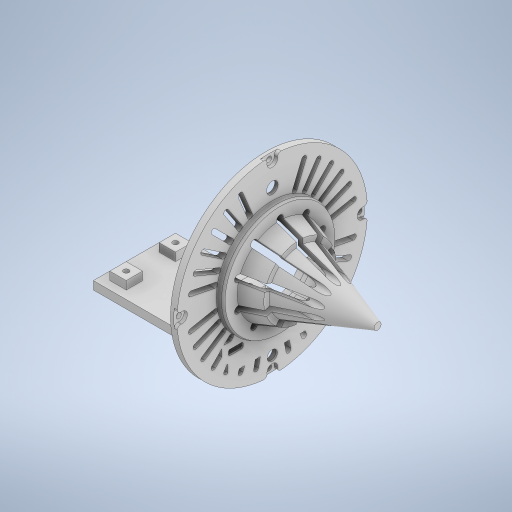
# Autodesk Inventor part: Temp_controller_trent_back
Saved by Autodesk Inventor 2024 (Build 280153000, 153)
## iProperties
Created: 2026-04-14
Part Number: Temp_controller_trent_back
Material: Generic
Document SubType Name: Modeling
Designer: Péter
Density: 1 g/cm^3
Appearance: Default
Author: Péter
Autodesk Inventor part; units mm, degrees
ref_plane "YZ Plane" through (0, 0, 0) normal (1, 0, 0) x (0, 1, 0)
ref_plane "XZ Plane" through (0, 0, 0) normal (0, 1, 0) x (-1, 0, 0)
ref_plane "XY Plane" through (0, 0, 0) normal (0, 0, 1) x (1, 0, 0)
sketch "Sketch1" plane through (0, 0, 0) normal (1, 0, 0) x (0, 1, 0)
  circle A0 centre (0, 0) radius 58
  dimension "d0" = 116
  constraints: 1 centre point, 1 coincident
  measures "d0" diameter of A0
extrude "Extrusion1" add sketch "Sketch1" along normal blind 4
sketch "Sketch2" plane through (0, 0, 0) normal (-1, 0, 0) x (0, 0, 1)
  line L0 (-25, -37.5) -> (25, -37.5)
  line L1 (25, -37.5) -> (25, -42.5)
  line L2 (25, -42.5) -> (-25, -42.5)
  line L3 (-25, -42.5) -> (-25, -37.5)
  line L4 (-25, -37.5) -> (25, -42.5) construction
  line L5 (25, -37.5) -> (-25, -42.5) construction
  point P0 (0, 0)
  point P1 (0, -40)
  dimension "d3" = 50
  dimension "d4" = 5
  dimension "d5" = 0
  dimension "d6" = 40
  constraints: 12 end point, 2 midpoint, 2 parallel, 1 horizontal, 1 perpendicular
  measures "d3" distance of L1.end L2.end
  measures "d4" distance of L0.end L1.end
  measures "d5" horizontal distance of point (0, 0) point (0, -40)
  measures "d6" distance of point (0, 0) point (0, -40)
extrude "Extrusion2" add sketch "Sketch2" along normal blind 80
sketch "Sketch3" plane through (0, -37.5, 25) normal (0, 1, 0) x (1, 0, 0)
  line L0 (-20, 45) -> (-30, 45)
  line L1 (-30, 45) -> (-30, 35)
  line L2 (-30, 35) -> (-20, 35)
  line L3 (-20, 35) -> (-20, 45)
  line L4 (-20, 45) -> (-30, 35) construction
  line L5 (-30, 45) -> (-20, 35) construction
  line L6 (-20, 15) -> (-30, 15)
  line L7 (-30, 15) -> (-30, 5)
  line L8 (-30, 5) -> (-20, 5)
  line L9 (-20, 5) -> (-20, 15)
  line L10 (-20, 15) -> (-30, 5) construction
  line L11 (-30, 15) -> (-20, 5) construction
  line L12 (-75, 35) -> (-65, 35)
  line L13 (-65, 35) -> (-65, 45)
  line L14 (-65, 45) -> (-75, 45)
  line L15 (-75, 45) -> (-75, 35)
  line L16 (-75, 35) -> (-65, 45) construction
  line L17 (-65, 35) -> (-75, 45) construction
  line L18 (-75, 15) -> (-65, 15)
  line L19 (-65, 15) -> (-65, 5)
  line L20 (-65, 5) -> (-75, 5)
  line L21 (-75, 5) -> (-75, 15)
  line L22 (-75, 15) -> (-65, 5) construction
  line L23 (-65, 15) -> (-75, 5) construction
  line L24 (-25, 40) -> (-70, 40) construction
  line L25 (-70, 40) -> (-70, 10) construction
  line L26 (-25, 10) -> (-70, 10) construction
  line L27 (-25, 10) -> (-25, 40) construction
  line L28 (0, 50) -> (0, 0) projected
  line L29 (0, 50) -> (-80, 50) projected
  line L30 (-80, 0) -> (-80, 50) projected
  point P0 (0, 25)
  point P1 (-80, 25)
  dimension "d9" = 10
  dimension "d10" = 10
  dimension "d11" = 10
  dimension "d12" = 10
  dimension "d13" = 10
  dimension "d14" = 10
  dimension "d15" = 10
  dimension "d16" = 10
  dimension "d17" = 30
  dimension "d18" = 45
  dimension "d19" = 15
  dimension "d20" = 10
  constraints: 56 end point, 12 parallel, 9 midpoint, 5 horizontal, 5 perpendicular
  measures "d9" distance of L2.end L1.end
  measures "d10" distance of L1.end L0.end
  measures "d11" distance of L8.end L7.end
  measures "d12" distance of L7.end L6.end
  measures "d13" distance of L14.end L13.end
  measures "d14" distance of L13.end L12.end
  measures "d15" distance of L19.end L20.end
  measures "d16" distance of L18.end L19.end
  measures "d17" distance of L24.end L25.end
  measures "d18" distance of L24.start L24.end
  measures "d19" distance from line of point (-80, 25) L24
  measures "d20" distance between parallel lines of L30 L25
extrude "Extrusion3" add sketch "Sketch3" along normal blind 5
sketch "Sketch4" plane through (0, -32.5, 25) normal (0, 1, 0) x (1, 0, 0)
  line L0 (-25, 10) -> (-25, 40) construction
  line L1 (-25, 40) -> (-70, 40) construction
  line L2 (-70, 40) -> (-70, 10) construction
  line L3 (-70, 10) -> (-25, 10) construction
  line L4 (0, 50) -> (-80, 50) projected
  line L5 (-80, 0) -> (-80, 50) projected
  line L6 (-75, 15) -> (-75, 5) projected
  line L7 (-75, 5) -> (-65, 5) projected
  point P0 (0, 25)
  dimension "d23" = 45
  dimension "d24" = 30
  dimension "d25" = 5
  dimension "d26" = 5
  constraints: 8 end point, 4 parallel, 1 vertical
  measures "d23" distance of L0.end L1.end
  measures "d24" distance of L1.end L2.end
  measures "d25" distance between parallel lines of L6 L2
  measures "d26" distance between parallel lines of L7 L3
hole "Hole1" at (-25, -32.5, -15) at (-25, -32.5, 15) at (-70, -32.5, 15) at (-70, -32.5, -15) direction (0, -1, 0) diameter 3.2 end through all
sketch "Sketch5" plane through (0, -42.5, -25) normal (0, -1, 0) x (1, 0, 0)
  circle A0 centre (-70, 40) radius 1.6 projected
  line L0 (-68.3834, 37.2) -> (-71.6166, 37.2)
  line L1 (-71.6166, 37.2) -> (-73.2332, 40)
  line L2 (-73.2332, 40) -> (-71.6166, 42.8)
  line L3 (-71.6166, 42.8) -> (-68.3834, 42.8)
  line L4 (-68.3834, 42.8) -> (-66.7668, 40)
  line L5 (-66.7668, 40) -> (-68.3834, 37.2)
  circle A1 centre (-70, 10) radius 1.6 projected
  line L6 (-68.3834, 7.2) -> (-71.6166, 7.2)
  line L7 (-71.6166, 7.2) -> (-73.2332, 10)
  line L8 (-73.2332, 10) -> (-71.6166, 12.8)
  line L9 (-71.6166, 12.8) -> (-68.3834, 12.8)
  line L10 (-68.3834, 12.8) -> (-66.7668, 10)
  line L11 (-66.7668, 10) -> (-68.3834, 7.2)
  line L12 (0, 50) -> (-80, 50) projected
  line L13 (0, 0) -> (-80, 0) projected
  line L14 (-23.3834, 37.2) -> (-26.6166, 37.2)
  line L15 (-26.6166, 37.2) -> (-28.2332, 40)
  line L16 (-28.2332, 40) -> (-26.6166, 42.8)
  line L17 (-26.6166, 42.8) -> (-23.3834, 42.8)
  line L18 (-23.3834, 42.8) -> (-21.7668, 40)
  line L19 (-21.7668, 40) -> (-23.3834, 37.2)
  circle A2 centre (-25, 10) radius 1.6 projected
  line L20 (-23.3834, 12.8) -> (-21.7668, 10)
  line L21 (-21.7668, 10) -> (-23.3834, 7.2)
  line L22 (-23.3834, 7.2) -> (-26.6166, 7.2)
  line L23 (-26.6166, 7.2) -> (-28.2332, 10)
  line L24 (-28.2332, 10) -> (-26.6166, 12.8)
  line L25 (-26.6166, 12.8) -> (-23.3834, 12.8)
  point P0 (0, 25)
  point P1 (-70, 40)
  point P2 (-70, 10)
  point P3 (-25, 40)
  point P4 (-25, 10)
  point P5 (-25, 37.2)
  dimension "d34" = 5.6
  dimension "d35" = 5.6
  dimension "d36" = 5.6
  dimension "d37" = 5.6
  constraints: 48 end point, 4 parallel, 3 coincident, 1 midpoint, 52 other
  measures "d34" distance from line of point (-25, 37.2) L17
  measures "d35" distance between parallel lines of L3 L0
  measures "d36" distance between parallel lines of L6 L9
  measures "d37" distance between parallel lines of L22 L25
extrude "Extrusion4" cut sketch "Sketch5" against normal blind 5
sketch "Sketch6" plane through (0, 0, 0) normal (0, 0, 1) x (1, 0, 0)
  line L0 (4, -58) -> (4, 58) projected
  line L1 (4, 34.1056) -> (7.1617, 34.1056)
  line L2 (7.1617, 34.1056) -> (8.6675, 33.4211)
  line L3 (8.6675, 33.4211) -> (8.6675, 26.0286)
  line L4 (8.6675, 26.0286) -> (20.6939, 21.84)
  line L5 (20.6939, 21.84) -> (20.6939, 18.6633)
  line L6 (20.6939, 18.6633) -> (68.159, 2.1319)
  line L7 (68.159, 2.1319) -> (68.159, 0)
  line L8 (68.159, 0) -> (65.159, 0)
  line L9 (65.159, 0) -> (17.6939, 16.5314)
  line L10 (17.6939, 16.5314) -> (17.6939, 19.7081)
  line L11 (17.6939, 19.7081) -> (6.6667, 23.5487)
  line L12 (6.6667, 23.5487) -> (4, 23.5487)
  line L13 (-109.6318, 0) -> (97.7908, 0) projected
  line L14 (59.0379, 2.1319) -> (59.0379, 0)
  line L15 (65.159, 0) -> (59.0379, 0)
  point P0 (0, 0)
  point P1 (20.6939, 20.2516)
  dimension "d53" = 0
  dimension "d54" = 3
  dimension "d55" = 3
  dimension "d56" = 3
  dimension "d57" = 3
  constraints: 28 end point, 6 parallel, 6 point on line, 3 perpendicular, 1 horizontal, 1 midpoint
  measures "d53" distance from line of point (0, 0) L8
  measures "d54" distance between parallel lines of L4 L11
  measures "d55" distance from line of point (20.694, 20.252) L10
  measures "d56" distance between parallel lines of L9 L6
  measures "d57" distance from line of L8.end L7
revolve "Revolution1" add sketch "Sketch6" angle 360 about axis through (-10, 0, 0) along (1, 0, 0) contours L0 L1 L2 L3 L4 L5 L6 L7 L8 L9 L10 L11 L12 | L14 L9 L13
sketch "Sketch7" plane through (0, 0, 0) normal (-1, 0, 0) x (0, 0, 1)
  circle A0 centre (0, 0) radius 23.5
  dimension "d59" = 47
  constraints: 1 centre point, 1 coincident
  measures "d59" diameter of A0
extrude "Extrusion5" cut sketch "Sketch7" against normal up to surface (4 mm away)
sketch "Sketch9" plane through (68.159, 0, 0) normal (1, 0, 0) x (0, 0, -1)
  line L0 (0, 27) -> (0, 12) construction
  line L1 (-2, 27) -> (-2, 12)
  line L2 (2, 12) -> (2, 27)
  arc A0 (2, 27) -> (-2, 27) centre (0, 27) ccw
  arc A1 (-2, 12) -> (2, 12) centre (0, 12) ccw
  line L3 (-15.8702, 21.8435) -> (-7.0534, 9.7082) construction
  line L4 (-17.4882, 20.6679) -> (-8.6715, 8.5326)
  line L5 (-5.4354, 10.8838) -> (-14.2522, 23.019)
  arc A2 (-14.2522, 23.019) -> (-17.4882, 20.6679) centre (-15.8702, 21.8435) ccw
  arc A3 (-8.6715, 8.5326) -> (-5.4354, 10.8838) centre (-7.0534, 9.7082) ccw
  line L6 (-25.6785, 8.3435) -> (-11.4127, 3.7082) construction
  line L7 (-26.2966, 6.4413) -> (-12.0307, 1.8061)
  line L8 (-10.7946, 5.6103) -> (-25.0605, 10.2456)
  arc A4 (-25.0605, 10.2456) -> (-26.2966, 6.4413) centre (-25.6785, 8.3435) ccw
  arc A5 (-12.0307, 1.8061) -> (-10.7946, 5.6103) centre (-11.4127, 3.7082) ccw
  line L9 (-25.6785, -8.3435) -> (-11.4127, -3.7082) construction
  line L10 (-25.0605, -10.2456) -> (-10.7946, -5.6103)
  line L11 (-12.0307, -1.8061) -> (-26.2966, -6.4413)
  arc A6 (-26.2966, -6.4413) -> (-25.0605, -10.2456) centre (-25.6785, -8.3435) ccw
  arc A7 (-10.7946, -5.6103) -> (-12.0307, -1.8061) centre (-11.4127, -3.7082) ccw
  line L12 (-15.8702, -21.8435) -> (-7.0534, -9.7082) construction
  line L13 (-14.2522, -23.019) -> (-5.4354, -10.8838)
  line L14 (-8.6715, -8.5326) -> (-17.4882, -20.6679)
  arc A8 (-17.4882, -20.6679) -> (-14.2522, -23.019) centre (-15.8702, -21.8435) ccw
  arc A9 (-5.4354, -10.8838) -> (-8.6715, -8.5326) centre (-7.0534, -9.7082) ccw
  line L15 (0, -27) -> (0, -12) construction
  line L16 (2, -27) -> (2, -12)
  line L17 (-2, -12) -> (-2, -27)
  arc A10 (-2, -27) -> (2, -27) centre (0, -27) ccw
  arc A11 (2, -12) -> (-2, -12) centre (0, -12) ccw
  line L18 (15.8702, -21.8435) -> (7.0534, -9.7082) construction
  line L19 (17.4882, -20.6679) -> (8.6715, -8.5326)
  line L20 (5.4354, -10.8838) -> (14.2522, -23.019)
  arc A12 (14.2522, -23.019) -> (17.4882, -20.6679) centre (15.8702, -21.8435) ccw
  arc A13 (8.6715, -8.5326) -> (5.4354, -10.8838) centre (7.0534, -9.7082) ccw
  line L21 (25.6785, -8.3435) -> (11.4127, -3.7082) construction
  line L22 (26.2966, -6.4413) -> (12.0307, -1.8061)
  line L23 (10.7946, -5.6103) -> (25.0605, -10.2456)
  arc A14 (25.0605, -10.2456) -> (26.2966, -6.4413) centre (25.6785, -8.3435) ccw
  arc A15 (12.0307, -1.8061) -> (10.7946, -5.6103) centre (11.4127, -3.7082) ccw
  line L24 (25.6785, 8.3435) -> (11.4127, 3.7082) construction
  line L25 (25.0605, 10.2456) -> (10.7946, 5.6103)
  line L26 (12.0307, 1.8061) -> (26.2966, 6.4413)
  arc A16 (26.2966, 6.4413) -> (25.0605, 10.2456) centre (25.6785, 8.3435) ccw
  arc A17 (10.7946, 5.6103) -> (12.0307, 1.8061) centre (11.4127, 3.7082) ccw
  line L27 (15.8702, 21.8435) -> (7.0534, 9.7082) construction
  line L28 (14.2522, 23.019) -> (5.4354, 10.8838)
  line L29 (8.6715, 8.5326) -> (17.4882, 20.6679)
  arc A18 (17.4882, 20.6679) -> (14.2522, 23.019) centre (15.8702, 21.8435) ccw
  arc A19 (5.4354, 10.8838) -> (8.6715, 8.5326) centre (7.0534, 9.7082) ccw
  point P0 (0, 0)
  point P1 (0, 19.5)
  point P2 (-11.4618, 15.7758)
  point P3 (-18.5456, 6.0258)
  point P4 (-18.5456, -6.0258)
  point P5 (-11.4618, -15.7758)
  point P6 (0, -19.5)
  point P7 (11.4618, -15.7758)
  point P8 (18.5456, -6.0258)
  point P9 (18.5456, 6.0258)
  point P10 (11.4618, 15.7758)
  dimension "d70" = 15
  dimension "d71" = 4
  dimension "d72" = 12
  dimension "d75" = 360
  constraints: 80 end point, 40 point on circle, 20 centre point, 4 tangent, 1 midpoint, 1 parallel, 1 vertical, 121 other
  measures "d70" distance of L0.start L0.end
  measures "d71" diameter of A1
  measures "d72" distance of point (0, 0) L0.end
extrude "Extrusion7" cut sketch "Sketch9" against normal up to surface (68.159 mm away)
sketch "Sketch10" plane through (4, 0, 0) normal (1, 0, 0) x (0, 0, -1)
  point P0 (0, 0)
  point P1 (0, -55)
  dimension "d79" = 55
  measures "d79" distance of point (0, 0) point (0, -55)
hole "Hole2" at (4, -55, 0) direction (-1, 0, 0) diameter 3.2 end through all
pattern_circular "Circular Pattern1" count 4 over 360 about axis through (5.5808, 0, 0) along (1, 0, 0) of "Hole2"
sketch "Sketch11" plane through (0, 0, 0) normal (-1, 0, 0) x (0, 0, 1)
  line L0 (-32.5, -29.5) -> (-12, -29.5)
  line L1 (-12, -29.5) -> (-12, -36.5)
  line L2 (-12, -36.5) -> (-32.5, -36.5)
  line L3 (-32.5, -36.5) -> (-32.5, -29.5)
  line L4 (-25, -37.5) -> (25, -37.5) projected
  point P0 (0, 0)
  dimension "d90" = 20.5
  dimension "d91" = 7
  dimension "d92" = 12
  dimension "d107" = 1
  constraints: 8 end point, 2 parallel, 1 horizontal, 1 perpendicular
  measures "d90" distance of L0.start L0.end
  measures "d91" distance of L2.end L0.start
  measures "d92" distance from line of point (0, 0) L1
  measures "d107" distance between parallel lines of L4 L2
extrude "Extrusion8" cut sketch "Sketch11" against normal blind 3
sketch "Sketch12" plane through (3, 0, 0) normal (-1, 0, 0) x (0, 0, 1)
  line L0 (-14.25, -33) -> (-30.25, -33) construction
  line L1 (-32.5, -29.5) -> (-12, -29.5) projected
  point P0 (0, 0)
  point P1 (-22.25, -29.5)
  point P2 (-22.25, -33)
  dimension "d96" = 16
  dimension "d97" = 3.5
  dimension "d98" = 0
  constraints: 2 end point, 2 midpoint, 1 parallel
  measures "d96" distance of L0.start L0.end
  measures "d97" distance between parallel lines of L1 L0
  measures "d98" horizontal distance of point (-22.25, -29.5) point (-22.25, -33)
hole "Hole3" at (3, -33, -30.25) at (3, -33, -14.25) direction (1, 0, 0) diameter 2.1 end through all
sketch "Sketch13" plane through (3, 0, 0) normal (-1, 0, 0) x (0, 0, 1)
  line L0 (-25.75, -31.35) -> (-18.75, -31.35)
  line L1 (-17.75, -32.35) -> (-17.75, -33.65)
  line L2 (-18.75, -34.65) -> (-25.75, -34.65)
  line L3 (-26.75, -33.65) -> (-26.75, -32.35)
  circle A0 centre (-30.25, -33) radius 1.05 projected
  arc A1 (-25.75, -31.35) -> (-26.75, -32.35) centre (-25.75, -32.35) ccw
  arc A2 (-26.75, -33.65) -> (-25.75, -34.65) centre (-25.75, -33.65) ccw
  arc A3 (-17.75, -32.35) -> (-18.75, -31.35) centre (-18.75, -32.35) ccw
  arc A4 (-18.75, -34.65) -> (-17.75, -33.65) centre (-18.75, -33.65) ccw
  point P0 (0, 0)
  point P1 (-17.75, -34.65)
  point P2 (-17.75, -31.35)
  point P3 (-26.75, -34.65)
  point P4 (-22.25, -34.65)
  point P5 (-26.75, -33)
  dimension "d108" = 9
  dimension "d109" = 3.3
  dimension "d110" = 8
  dimension "d111" = 0
  dimension "d112" = 1
  dimension "d113" = 1
  constraints: 8 end point, 8 point on circle, 8 tangent, 6 point on line, 4 centre point, 2 equal radius, 2 midpoint, 2 parallel, 1 horizontal, 1 perpendicular
  measures "d108" distance of point (-17.75, -34.65) point (-26.75, -34.65)
  measures "d109" distance of point (-17.75, -31.35) point (-17.75, -34.65)
  measures "d110" horizontal distance of A0.centre point (-22.25, -34.65)
  measures "d111" vertical distance of point (-26.75, -33) A0.centre
  measures "d112" radius of A1
  measures "d113" radius of A2
extrude "Extrusion9" cut sketch "Sketch13" against normal up to surface (1 mm away) contours L0 A3 L1 A4 L2 A2 L3 A1
mirror "Mirror1" about plane through (0, 0, 0) normal (0, 0, 1) of "Extrusion9"
sketch "Sketch14" plane through (3, -33.65, 17.75) normal (1, 0, 0) x (0, 0, -1)
  line L0 (-8, 2.3) -> (-1, 2.3)
  line L1 (0, 1.3) -> (0, 0)
  line L2 (-1, -1) -> (-8, -1)
  line L3 (-9, 0) -> (-9, 1.3)
  line L4 (-8, 2.3) -> (-1, 2.3) projected
  line L5 (-9, 0) -> (-9, 1.3) projected
  line L6 (0, 1.3) -> (0, 0) projected
  line L7 (-1, -1) -> (-8, -1) projected
  arc A0 (-8, 2.3) -> (-9, 1.3) centre (-8, 1.3) ccw
  arc A1 (-9, 0) -> (-8, -1) centre (-8, 0) ccw
  arc A2 (-1, -1) -> (0, 0) centre (-1, 0) ccw
  arc A3 (0, 1.3) -> (-1, 2.3) centre (-1, 1.3) ccw
  point P0 (17.75, 33.65)
  dimension "d116" = 1
  constraints: 8 end point, 8 point on circle, 8 tangent, 4 centre point, 4 collinear, 3 equal radius, 2 parallel, 1 horizontal, 1 perpendicular
  measures "d116" radius of A0
extrude "Extrusion10" cut sketch "Sketch14" against normal up to surface (3 mm away)
sketch "Sketch15" plane through (0, 0, 0) normal (-1, 0, 0) x (0, 0, 1)
  line L0 (15.75, -29.35) -> (28.75, -29.35)
  line L1 (28.75, -29.35) -> (28.75, -36.65)
  line L2 (28.75, -36.65) -> (15.75, -36.65)
  line L3 (15.75, -36.65) -> (15.75, -29.35)
  line L4 (18.75, -31.35) -> (25.75, -31.35) projected
  line L5 (26.75, -32.35) -> (26.75, -33.65) projected
  line L6 (17.75, -33.65) -> (17.75, -32.35) projected
  line L7 (25.75, -34.65) -> (18.75, -34.65) projected
  point P0 (0, 0)
  point P1 (26.75, -33)
  point P2 (15.75, -33)
  dimension "d119" = 2
  dimension "d120" = 2
  dimension "d121" = 2
  dimension "d122" = 2
  constraints: 8 end point, 2 midpoint, 2 parallel, 1 horizontal, 1 perpendicular
  measures "d119" distance between parallel lines of L0 L4
  measures "d120" distance from line of point (26.75, -33) L1
  measures "d121" distance from line of point (15.75, -33) L6
  measures "d122" distance between parallel lines of L7 L2
extrude "Extrusion11" cut sketch "Sketch15" against normal blind 3
ref_plane "Work Plane1" through (4, -36.25, 25.75) normal (0, 1, 0) x (1, 0, 0)
sketch "Sketch16" plane through (4, -36.25, 25.75) normal (0, 1, 0) x (1, 0, 0)
  line L0 (-7, 0.75) -> (-10, 0.75)
  line L1 (-10, 0.75) -> (-10, 8.5)
  line L2 (-10, 8.5) -> (-7, 8.5)
  line L3 (-7, 8.5) -> (-7, 0.75)
  line L4 (-4, 50.75) -> (-4, 0.75) projected
  line L5 (-4, 10) -> (-1, 10) projected
  line L6 (-4, 0.75) -> (-84, 0.75) projected
  line L7 (-7, 0.75) -> (-10, 0.75)
  point P0 (-4, 25.75)
  dimension "d126" = 3
  dimension "d128" = 3
  dimension "d129" = 1.5
  constraints: 10 end point, 4 point on line, 2 parallel, 1 collinear, 1 horizontal, 1 perpendicular
  measures "d126" distance of L1.end L2.end
  measures "d128" distance between parallel lines of L4 L3
  measures "d129" distance between parallel lines of L5 L2
extrude "Extrusion12" add sketch "Sketch16" against normal up to surface (1.25 mm away)
sketch "Sketch18" plane through (0, 0, 0) normal (-1, 0, 0) x (0, 0, 1)
  circle A0 centre (0, -47.5) radius 4.25
  line L0 (25, -42.5) -> (-25, -42.5) projected
  point P0 (0, 0)
  dimension "d133" = 8.5
  dimension "d134" = 5
  constraints: 1 centre point
  measures "d133" diameter of A0
  measures "d134" distance from line of L0 A0.centre
extrude "Extrusion13" cut sketch "Sketch18" against normal blind 3
sketch "Sketch19" plane through (3, -47.5, 0) normal (-1, 0, 0) x (0, 0, 1)
  point P0 (0, 47.5)
  point P1 (0, 0)
hole "Hole4" at (3, -47.5, 0) direction (1, 0, 0) diameter 6.2 end through all
sketch "Sketch20" plane through (0, 0, 0) normal (-1, 0, 0) x (0, 0, 1)
  circle A0 centre (0, 55) radius 1.6 projected
  point P0 (0, 0)
  point P1 (0, 41)
  dimension "d144" = 14
  measures "d144" distance of A0.centre point (0, 41)
hole "Hole5" at (0, 41, 0) direction (1, 0, 0) diameter 7 end through all
sketch "Sketch21" plane through (0, 0, 0) normal (-1, 0, 0) x (0, 0, 1)
  line L0 (-7.5, 48.5) -> (7.5, 48.5)
  line L1 (7.5, 48.5) -> (7.5, 33.5)
  line L2 (7.5, 33.5) -> (-7.5, 33.5)
  line L3 (-7.5, 33.5) -> (-7.5, 48.5)
  circle A0 centre (0, 41) radius 3.5 projected
  line L4 (-7.5, 48.5) -> (7.5, 33.5) construction
  line L5 (7.5, 48.5) -> (-7.5, 33.5) construction
  point P0 (0, 0)
  dimension "d152" = 15
  dimension "d153" = 15
  constraints: 12 end point, 2 midpoint, 2 parallel, 1 horizontal, 1 perpendicular
  measures "d152" distance of L1.end L2.end
  measures "d153" distance of L0.end L1.end
extrude "Extrusion14" cut sketch "Sketch21" against normal blind 2
sketch "Sketch22" plane through (0, 0, 0) normal (-1, 0, 0) x (0, 0, 1)
  line L0 (-35.6056, 0) -> (-50.6056, 0) construction
  line L1 (-35.6056, 1.5) -> (-50.6056, 1.5)
  line L2 (-50.6056, -1.5) -> (-35.6056, -1.5)
  arc A0 (-35.6056, -1.5) -> (-35.6056, 1.5) centre (-35.6056, 0) ccw
  arc A1 (-50.6056, 1.5) -> (-50.6056, -1.5) centre (-50.6056, 0) ccw
  circle A2 centre (0, 0) radius 34.1056 projected
  line L3 (-34.9214, -6.9463) -> (-49.6332, -9.8727) construction
  line L4 (-35.2141, -5.4751) -> (-49.9259, -8.4015)
  line L5 (-49.3406, -11.3438) -> (-34.6288, -8.4175)
  arc A3 (-34.6288, -8.4175) -> (-35.2141, -5.4751) centre (-34.9214, -6.9463) ccw
  arc A4 (-49.9259, -8.4015) -> (-49.3406, -11.3438) centre (-49.6332, -9.8727) ccw
  line L6 (-32.8953, -13.6257) -> (-46.7535, -19.3659) construction
  line L7 (-33.4693, -12.2399) -> (-47.3275, -17.9801)
  line L8 (-46.1794, -20.7517) -> (-32.3213, -15.0115)
  arc A5 (-32.3213, -15.0115) -> (-33.4693, -12.2399) centre (-32.8953, -13.6257) ccw
  arc A6 (-47.3275, -17.9801) -> (-46.1794, -20.7517) centre (-46.7535, -19.3659) ccw
  line L9 (-29.605, -19.7814) -> (-42.077, -28.115) construction
  line L10 (-30.4383, -18.5342) -> (-42.9104, -26.8678)
  line L11 (-41.2437, -29.3622) -> (-28.7716, -21.0286)
  arc A7 (-28.7716, -21.0286) -> (-30.4383, -18.5342) centre (-29.605, -19.7814) ccw
  arc A8 (-42.9104, -26.8678) -> (-41.2437, -29.3622) centre (-42.077, -28.115) ccw
  line L12 (-25.177, -25.177) -> (-35.7836, -35.7836) construction
  line L13 (-26.2376, -24.1163) -> (-36.8442, -34.7229)
  line L14 (-34.7229, -36.8442) -> (-24.1163, -26.2376)
  arc A9 (-24.1163, -26.2376) -> (-26.2376, -24.1163) centre (-25.177, -25.177) ccw
  arc A10 (-36.8442, -34.7229) -> (-34.7229, -36.8442) centre (-35.7836, -35.7836) ccw
  line L15 (-19.7814, -29.605) -> (-28.115, -42.077) construction
  line L16 (-21.0286, -28.7716) -> (-29.3622, -41.2437)
  line L17 (-26.8678, -42.9104) -> (-18.5342, -30.4383)
  arc A11 (-18.5342, -30.4383) -> (-21.0286, -28.7716) centre (-19.7814, -29.605) ccw
  arc A12 (-29.3622, -41.2437) -> (-26.8678, -42.9104) centre (-28.115, -42.077) ccw
  line L18 (-13.6257, -32.8953) -> (-19.3659, -46.7535) construction
  line L19 (-15.0115, -32.3213) -> (-20.7517, -46.1794)
  line L20 (-17.9801, -47.3275) -> (-12.2399, -33.4693)
  arc A13 (-12.2399, -33.4693) -> (-15.0115, -32.3213) centre (-13.6257, -32.8953) ccw
  arc A14 (-20.7517, -46.1794) -> (-17.9801, -47.3275) centre (-19.3659, -46.7535) ccw
  line L21 (-6.9463, -34.9214) -> (-9.8727, -49.6332) construction
  line L22 (-8.4175, -34.6288) -> (-11.3438, -49.3406)
  line L23 (-8.4015, -49.9259) -> (-5.4751, -35.2141)
  arc A15 (-5.4751, -35.2141) -> (-8.4175, -34.6288) centre (-6.9463, -34.9214) ccw
  arc A16 (-11.3438, -49.3406) -> (-8.4015, -49.9259) centre (-9.8727, -49.6332) ccw
  line L24 (0, -35.6056) -> (0, -50.6056) construction
  line L25 (-1.5, -35.6056) -> (-1.5, -50.6056)
  line L26 (1.5, -50.6056) -> (1.5, -35.6056)
  arc A17 (1.5, -35.6056) -> (-1.5, -35.6056) centre (0, -35.6056) ccw
  arc A18 (-1.5, -50.6056) -> (1.5, -50.6056) centre (0, -50.6056) ccw
  line L27 (6.9463, -34.9214) -> (9.8727, -49.6332) construction
  line L28 (5.4751, -35.2141) -> (8.4015, -49.9259)
  line L29 (11.3438, -49.3406) -> (8.4175, -34.6288)
  arc A19 (8.4175, -34.6288) -> (5.4751, -35.2141) centre (6.9463, -34.9214) ccw
  arc A20 (8.4015, -49.9259) -> (11.3438, -49.3406) centre (9.8727, -49.6332) ccw
  line L30 (13.6257, -32.8953) -> (19.3659, -46.7535) construction
  line L31 (12.2399, -33.4693) -> (17.9801, -47.3275)
  line L32 (20.7517, -46.1794) -> (15.0115, -32.3213)
  arc A21 (15.0115, -32.3213) -> (12.2399, -33.4693) centre (13.6257, -32.8953) ccw
  arc A22 (17.9801, -47.3275) -> (20.7517, -46.1794) centre (19.3659, -46.7535) ccw
  line L33 (19.7814, -29.605) -> (28.115, -42.077) construction
  line L34 (18.5342, -30.4383) -> (26.8678, -42.9104)
  line L35 (29.3622, -41.2437) -> (21.0286, -28.7716)
  arc A23 (21.0286, -28.7716) -> (18.5342, -30.4383) centre (19.7814, -29.605) ccw
  arc A24 (26.8678, -42.9104) -> (29.3622, -41.2437) centre (28.115, -42.077) ccw
  line L36 (25.177, -25.177) -> (35.7836, -35.7836) construction
  line L37 (24.1163, -26.2376) -> (34.7229, -36.8442)
  line L38 (36.8442, -34.7229) -> (26.2376, -24.1163)
  arc A25 (26.2376, -24.1163) -> (24.1163, -26.2376) centre (25.177, -25.177) ccw
  arc A26 (34.7229, -36.8442) -> (36.8442, -34.7229) centre (35.7836, -35.7836) ccw
  line L39 (29.605, -19.7814) -> (42.077, -28.115) construction
  line L40 (28.7716, -21.0286) -> (41.2437, -29.3622)
  line L41 (42.9104, -26.8678) -> (30.4383, -18.5342)
  arc A27 (30.4383, -18.5342) -> (28.7716, -21.0286) centre (29.605, -19.7814) ccw
  arc A28 (41.2437, -29.3622) -> (42.9104, -26.8678) centre (42.077, -28.115) ccw
  line L42 (32.8953, -13.6257) -> (46.7535, -19.3659) construction
  line L43 (32.3213, -15.0115) -> (46.1794, -20.7517)
  line L44 (47.3275, -17.9801) -> (33.4693, -12.2399)
  arc A29 (33.4693, -12.2399) -> (32.3213, -15.0115) centre (32.8953, -13.6257) ccw
  arc A30 (46.1794, -20.7517) -> (47.3275, -17.9801) centre (46.7535, -19.3659) ccw
  line L45 (34.9214, -6.9463) -> (49.6332, -9.8727) construction
  line L46 (34.6288, -8.4175) -> (49.3406, -11.3438)
  line L47 (49.9259, -8.4015) -> (35.2141, -5.4751)
  arc A31 (35.2141, -5.4751) -> (34.6288, -8.4175) centre (34.9214, -6.9463) ccw
  arc A32 (49.3406, -11.3438) -> (49.9259, -8.4015) centre (49.6332, -9.8727) ccw
  line L48 (35.6056, 0) -> (50.6056, 0) construction
  line L49 (35.6056, -1.5) -> (50.6056, -1.5)
  line L50 (50.6056, 1.5) -> (35.6056, 1.5)
  arc A33 (35.6056, 1.5) -> (35.6056, -1.5) centre (35.6056, 0) ccw
  arc A34 (50.6056, -1.5) -> (50.6056, 1.5) centre (50.6056, 0) ccw
  line L51 (34.9214, 6.9463) -> (49.6332, 9.8727) construction
  line L52 (35.2141, 5.4751) -> (49.9259, 8.4015)
  line L53 (49.3406, 11.3438) -> (34.6288, 8.4175)
  arc A35 (34.6288, 8.4175) -> (35.2141, 5.4751) centre (34.9214, 6.9463) ccw
  arc A36 (49.9259, 8.4015) -> (49.3406, 11.3438) centre (49.6332, 9.8727) ccw
  line L54 (32.8953, 13.6257) -> (46.7535, 19.3659) construction
  line L55 (33.4693, 12.2399) -> (47.3275, 17.9801)
  line L56 (46.1794, 20.7517) -> (32.3213, 15.0115)
  arc A37 (32.3213, 15.0115) -> (33.4693, 12.2399) centre (32.8953, 13.6257) ccw
  arc A38 (47.3275, 17.9801) -> (46.1794, 20.7517) centre (46.7535, 19.3659) ccw
  line L57 (29.605, 19.7814) -> (42.077, 28.115) construction
  line L58 (30.4383, 18.5342) -> (42.9104, 26.8678)
  line L59 (41.2437, 29.3622) -> (28.7716, 21.0286)
  arc A39 (28.7716, 21.0286) -> (30.4383, 18.5342) centre (29.605, 19.7814) ccw
  arc A40 (42.9104, 26.8678) -> (41.2437, 29.3622) centre (42.077, 28.115) ccw
  line L60 (25.177, 25.177) -> (35.7836, 35.7836) construction
  line L61 (26.2376, 24.1163) -> (36.8442, 34.7229)
  line L62 (34.7229, 36.8442) -> (24.1163, 26.2376)
  arc A41 (24.1163, 26.2376) -> (26.2376, 24.1163) centre (25.177, 25.177) ccw
  arc A42 (36.8442, 34.7229) -> (34.7229, 36.8442) centre (35.7836, 35.7836) ccw
  line L63 (19.7814, 29.605) -> (28.115, 42.077) construction
  line L64 (21.0286, 28.7716) -> (29.3622, 41.2437)
  line L65 (26.8678, 42.9104) -> (18.5342, 30.4383)
  arc A43 (18.5342, 30.4383) -> (21.0286, 28.7716) centre (19.7814, 29.605) ccw
  arc A44 (29.3622, 41.2437) -> (26.8678, 42.9104) centre (28.115, 42.077) ccw
  line L66 (13.6257, 32.8953) -> (19.3659, 46.7535) construction
  line L67 (15.0115, 32.3213) -> (20.7517, 46.1794)
  line L68 (17.9801, 47.3275) -> (12.2399, 33.4693)
  arc A45 (12.2399, 33.4693) -> (15.0115, 32.3213) centre (13.6257, 32.8953) ccw
  arc A46 (20.7517, 46.1794) -> (17.9801, 47.3275) centre (19.3659, 46.7535) ccw
  line L69 (6.9463, 34.9214) -> (9.8727, 49.6332) construction
  line L70 (8.4175, 34.6288) -> (11.3438, 49.3406)
  line L71 (8.4015, 49.9259) -> (5.4751, 35.2141)
  arc A47 (5.4751, 35.2141) -> (8.4175, 34.6288) centre (6.9463, 34.9214) ccw
  arc A48 (11.3438, 49.3406) -> (8.4015, 49.9259) centre (9.8727, 49.6332) ccw
  line L72 (0, 35.6056) -> (0, 50.6056) construction
  line L73 (1.5, 35.6056) -> (1.5, 50.6056)
  line L74 (-1.5, 50.6056) -> (-1.5, 35.6056)
  arc A49 (-1.5, 35.6056) -> (1.5, 35.6056) centre (0, 35.6056) ccw
  arc A50 (1.5, 50.6056) -> (-1.5, 50.6056) centre (0, 50.6056) ccw
  line L75 (-6.9463, 34.9214) -> (-9.8727, 49.6332) construction
  line L76 (-5.4751, 35.2141) -> (-8.4015, 49.9259)
  line L77 (-11.3438, 49.3406) -> (-8.4175, 34.6288)
  arc A51 (-8.4175, 34.6288) -> (-5.4751, 35.2141) centre (-6.9463, 34.9214) ccw
  arc A52 (-8.4015, 49.9259) -> (-11.3438, 49.3406) centre (-9.8727, 49.6332) ccw
  line L78 (-13.6257, 32.8953) -> (-19.3659, 46.7535) construction
  line L79 (-12.2399, 33.4693) -> (-17.9801, 47.3275)
  line L80 (-20.7517, 46.1794) -> (-15.0115, 32.3213)
  arc A53 (-15.0115, 32.3213) -> (-12.2399, 33.4693) centre (-13.6257, 32.8953) ccw
  arc A54 (-17.9801, 47.3275) -> (-20.7517, 46.1794) centre (-19.3659, 46.7535) ccw
  line L81 (-19.7814, 29.605) -> (-28.115, 42.077) construction
  line L82 (-18.5342, 30.4383) -> (-26.8678, 42.9104)
  line L83 (-29.3622, 41.2437) -> (-21.0286, 28.7716)
  arc A55 (-21.0286, 28.7716) -> (-18.5342, 30.4383) centre (-19.7814, 29.605) ccw
  arc A56 (-26.8678, 42.9104) -> (-29.3622, 41.2437) centre (-28.115, 42.077) ccw
  line L84 (-25.177, 25.177) -> (-35.7836, 35.7836) construction
  line L85 (-24.1163, 26.2376) -> (-34.7229, 36.8442)
  line L86 (-36.8442, 34.7229) -> (-26.2376, 24.1163)
  arc A57 (-26.2376, 24.1163) -> (-24.1163, 26.2376) centre (-25.177, 25.177) ccw
  arc A58 (-34.7229, 36.8442) -> (-36.8442, 34.7229) centre (-35.7836, 35.7836) ccw
  line L87 (-29.605, 19.7814) -> (-42.077, 28.115) construction
  line L88 (-28.7716, 21.0286) -> (-41.2437, 29.3622)
  line L89 (-42.9104, 26.8678) -> (-30.4383, 18.5342)
  arc A59 (-30.4383, 18.5342) -> (-28.7716, 21.0286) centre (-29.605, 19.7814) ccw
  arc A60 (-41.2437, 29.3622) -> (-42.9104, 26.8678) centre (-42.077, 28.115) ccw
  line L90 (-32.8953, 13.6257) -> (-46.7535, 19.3659) construction
  line L91 (-32.3213, 15.0115) -> (-46.1794, 20.7517)
  line L92 (-47.3275, 17.9801) -> (-33.4693, 12.2399)
  arc A61 (-33.4693, 12.2399) -> (-32.3213, 15.0115) centre (-32.8953, 13.6257) ccw
  arc A62 (-46.1794, 20.7517) -> (-47.3275, 17.9801) centre (-46.7535, 19.3659) ccw
  line L93 (-34.9214, 6.9463) -> (-49.6332, 9.8727) construction
  line L94 (-34.6288, 8.4175) -> (-49.3406, 11.3438)
  line L95 (-49.9259, 8.4015) -> (-35.2141, 5.4751)
  arc A63 (-35.2141, 5.4751) -> (-34.6288, 8.4175) centre (-34.9214, 6.9463) ccw
  arc A64 (-49.3406, 11.3438) -> (-49.9259, 8.4015) centre (-49.6332, 9.8727) ccw
  line L96 (9, 32) -> (-9, 32)
  line L97 (-9, 32) -> (-9, 50)
  line L98 (-9, 50) -> (9, 50)
  line L99 (9, 50) -> (9, 32)
  circle A65 centre (0, 41) radius 3.5 projected
  line L100 (9, 32) -> (-9, 50) construction
  line L101 (-9, 32) -> (9, 50) construction
  line L102 (-34.5, -27.5) -> (-10, -27.5)
  line L103 (-10, -27.5) -> (-10, -38.5)
  line L104 (-10, -38.5) -> (-34.5, -38.5)
  line L105 (-34.5, -38.5) -> (-34.5, -27.5)
  line L106 (13.75, -27.35) -> (30.75, -27.35)
  line L107 (30.75, -27.35) -> (30.75, -38.65)
  line L108 (30.75, -38.65) -> (13.75, -38.65)
  line L109 (13.75, -38.65) -> (13.75, -27.35)
  line L110 (-27, -35.5) -> (27, -35.5)
  line L111 (27, -35.5) -> (27, -44.5)
  line L112 (27, -44.5) -> (-27, -44.5)
  line L113 (-27, -44.5) -> (-27, -35.5)
  line L114 (-25, -42.5) -> (25, -42.5) projected
  line L115 (25, -37.5) -> (-25, -37.5) projected
  line L116 (25, -42.5) -> (25, -37.5) projected
  line L117 (-25, -37.5) -> (-25, -42.5) projected
  line L118 (28.75, -36.65) -> (15.75, -36.65) projected
  line L119 (28.75, -29.35) -> (28.75, -36.65) projected
  line L120 (15.75, -29.35) -> (28.75, -29.35) projected
  line L121 (15.75, -36.65) -> (15.75, -29.35) projected
  line L122 (-12, -29.5) -> (-12, -36.5) projected
  line L123 (-32.5, -29.5) -> (-12, -29.5) projected
  line L124 (-32.5, -36.5) -> (-32.5, -29.5) projected
  line L125 (-12, -36.5) -> (-32.5, -36.5) projected
  circle A66 centre (0, -47.5) radius 4.25 projected
  circle A67 centre (0, -47.5) radius 5.9
  circle A68 centre (0, -55) radius 1.6 projected
  circle A69 centre (55, 0) radius 1.6 projected
  point P0 (-43.1056, 0)
  point P1 (-42.2773, -8.4095)
  point P2 (-39.8244, -16.4958)
  point P3 (-35.841, -23.9482)
  point P4 (-30.4803, -30.4803)
  point P5 (-23.9482, -35.841)
  point P6 (-16.4958, -39.8244)
  point P7 (-8.4095, -42.2773)
  point P8 (0, -43.1056)
  point P9 (8.4095, -42.2773)
  point P10 (16.4958, -39.8244)
  point P11 (23.9482, -35.841)
  point P12 (30.4803, -30.4803)
  point P13 (35.841, -23.9482)
  point P14 (39.8244, -16.4958)
  point P15 (42.2773, -8.4095)
  point P16 (43.1056, 0)
  point P17 (42.2773, 8.4095)
  point P18 (39.8244, 16.4958)
  point P19 (35.841, 23.9482)
  point P20 (30.4803, 30.4803)
  point P21 (23.9482, 35.841)
  point P22 (16.4958, 39.8244)
  point P23 (8.4095, 42.2773)
  point P24 (0, 43.1056)
  point P25 (-8.4095, 42.2773)
  point P26 (-16.4958, 39.8244)
  point P27 (-23.9482, 35.841)
  point P28 (-30.4803, 30.4803)
  point P29 (-35.841, 23.9482)
  point P30 (-39.8244, 16.4958)
  point P31 (-42.2773, 8.4095)
  point P32 (13.081, -35.5)
  point P33 (13.75, -35.5)
  point P34 (13.75, -31.4004)
  point P35 (5.532, -35.5)
  point P36 (8.5908, -35.5)
  point P37 (-1.4963, -35.5)
  point P38 (1.4963, -35.5)
  point P39 (-8.5908, -35.5)
  point P40 (-5.532, -35.5)
  point P41 (-29.6213, -27.5)
  point P42 (-25.3787, -27.5)
  point P43 (-34.5, -36.6213)
  point P44 (-34.5, -32.3787)
  point P45 (-27, -43.0804)
  point P46 (-27, -38.5)
  point P47 (-27.5289, -38.5)
  point P48 (-16.8089, -44.5)
  point P49 (-20.0561, -44.5)
  point P50 (-7.3222, -44.5)
  point P51 (-10.381, -44.5)
  point P52 (10.381, -44.5)
  point P53 (7.3222, -44.5)
  point P54 (20.0561, -44.5)
  point P55 (16.8089, -44.5)
  point P56 (27, -38.65)
  point P57 (27, -43.0804)
  point P58 (27.6291, -38.65)
  point P59 (30.75, -28.6287)
  point P60 (30.75, -32.8713)
  point P61 (25.2287, -27.35)
  point P62 (29.4713, -27.35)
  point P63 (9, 37.5573)
  point P64 (8.4182, 50)
  point P65 (-1.5, 50)
  point P66 (1.5, 50)
  point P67 (-8.4182, 50)
  point P68 (-9, 37.5573)
  dimension "d156" = 15
  dimension "d157" = 3
  dimension "d160" = 360
  dimension "d162" = 18
  dimension "d163" = 18
  dimension "d164" = 2
  dimension "d165" = 2
  dimension "d166" = 2
  dimension "d167" = 2
  dimension "d168" = 2
  dimension "d169" = 2
  dimension "d170" = 2
  dimension "d171" = 2
  dimension "d172" = 2
  dimension "d173" = 2
  dimension "d174" = 2
  dimension "d175" = 2
  constraints: 292 end point, 128 point on circle, 65 centre point, 9 parallel, 6 tangent, 5 horizontal, 4 perpendicular, 3 midpoint, 1 coincident, 385 other
  measures "d156" distance of L0.start L0.end
  measures "d157" diameter of A1
  measures "d162" distance of L97.end L98.end
  measures "d163" distance of L96.end L97.end
  measures "d164" distance between parallel lines of L114 L112
  measures "d165" distance between parallel lines of L115 L110
  measures "d166" distance between parallel lines of L116 L111
  measures "d167" distance between parallel lines of L117 L113
  measures "d168" distance between parallel lines of L118 L108
  measures "d169" distance between parallel lines of L119 L107
  measures "d170" distance between parallel lines of L106 L120
  measures "d171" distance between parallel lines of L109 L121
  measures "d172" distance between parallel lines of L103 L122
  measures "d173" distance between parallel lines of L102 L123
  measures "d174" distance between parallel lines of L124 L105
  measures "d175" distance between parallel lines of L125 L104
extrude "Extrusion15" cut sketch "Sketch22" against normal up to surface (4 mm away) contours A63 L95 A64 L94 | A61 L92 A62 L91 | A59 L89 A60 L88 | A57 L86 A58 L85 | A55 L83 A56 L82 | A53 L80 A54 L79 | A45 L68 A46 L67 | A43 L65 A44 L64 | A41 L62 A42 L61 | A39 L59 A40 L58 | A37 L56 A38 L55 | A35 L53 A36 L52 | A31 L47 A32 L46 | A29 L44 A30 L43 | A27 L41 A28 L40 | A7 L11 A8 L10 | A5 L8 A6 L7 | A3 L5 A4 L4 | A9 L14 L102 L13 | A15 L23 L110 L22 | L105 L14 A10 L13 | A17 L110 | A19 L29 L110 L28 | L104 L113 A12 L16 | L112 L23 A16 L22 | L20 A14 L19 L112 | L112 L29 A20 L28 | A25 L38 L106 L37 | L112 L32 A22 L31 | L38 A26 L37 L107 | L111 L108 L35 A24
sketch "Sketch23" plane through (4, 0, 0) normal (1, 0, 0) x (0, 0, -1)
  circle A0 centre (-55, 0) radius 1.6 projected
  circle A1 centre (-55, 0) radius 3.25
  circle A2 centre (0, 55) radius 1.6 projected
  circle A3 centre (0, 55) radius 3.25
  circle A4 centre (55, 0) radius 1.6 projected
  circle A5 centre (55, 0) radius 3.25
  circle A6 centre (0, -55) radius 1.6 projected
  circle A7 centre (0, -55) radius 3.25
  point P0 (0, 0)
  dimension "d178" = 6.5
  dimension "d179" = 6.5
  dimension "d180" = 6.5
  dimension "d181" = 6.5
  constraints: 4 centre point, 4 coincident
  measures "d178" diameter of A1
  measures "d179" diameter of A3
  measures "d180" diameter of A5
  measures "d181" diameter of A7
extrude "Extrusion16" cut sketch "Sketch23" against normal blind 2 contours A0 | A1 | A2 | A3 | A4 | A5 | A6 | A7
fillet "Fillet1" radius 2 8 edges at (3, 1.2836, 57.9858) (3, -1.2836, 57.9858) (3, 1.2836, -57.9858) (3, -1.2836, -57.9858) (3, -57.9858, -1.2836) (3, -57.9858, 1.2836) (3, 57.9858, 1.2836) (3, 57.9858, -1.2836)
body "Solid1"
